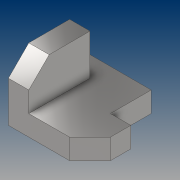
# Autodesk Inventor part: 10
Saved by Autodesk Inventor 2020.2 (Build 242310000, 310)
## iProperties
Created: 2020-09-17
Part Number: 10
Material: 鋼、碳鋼
Document SubType Name: Modeling
Designer: user
Density: 7.85 g/cm^3
Appearance: 半拋光
Mass: 149.15 g
Surface Area: 56.8284 cm^2
Volume: 19 cm^3
Author: user
Autodesk Inventor part; units mm, degrees
ref_plane "YZ Plane" through (0, 0, 0) normal (1, 0, 0) x (0, 1, 0)
ref_plane "XZ Plane" through (0, 0, 0) normal (0, 1, 0) x (-1, 0, 0)
ref_plane "XY Plane" through (0, 0, 0) normal (0, 0, 1) x (1, 0, 0)
sketch "草圖1" plane through (0, 0, 0) normal (0, 1, 0) x (-1, 0, 0)
  line L0 (0, 0) -> (-40, 0)
  line L1 (-40, 0) -> (-40, 40)
  line L2 (-40, 40) -> (0, 40)
  line L3 (0, 40) -> (0, 0)
  line L4 (-30, 0) -> (-30, 20)
  line L5 (-30, 20) -> (-40, 20)
  line L6 (-30, 40) -> (-40, 30)
  dimension "d0" = 40
  dimension "d1" = 40
  dimension "d2" = 10
  dimension "d3" = 20
  dimension "d4" = 10
  dimension "d5" = 10
  constraints: 14 end point, 3 point on line, 2 parallel, 2 perpendicular, 1 horizontal, 1 midpoint, 1 vertical
  measures "d0" distance of L0.start L0.end
  measures "d1" distance of L2.end L0.start
  measures "d2" distance between parallel lines of L1 L4
  measures "d3" distance of L4.start L4.end
  measures "d4" distance from line of L2 L6.end
  measures "d5" distance from line of L6.start L1
extrude "擠出1" add sketch "草圖1" along normal blind 10 contours L0 L4 L5 L1 L6 L2 L3
sketch "草圖2" plane through (0, 0, 0) normal (-1, 0, 0) x (0, 0, 1)
  line L0 (40, 10) -> (40, 0) projected
  line L1 (40, 0) -> (0, 0) projected
  line L2 (0, 0) -> (0, 10) projected
  line L3 (0, 10) -> (40, 10) projected
  line L4 (40, 10) -> (40, 20)
  line L5 (40, 20) -> (30, 30)
  line L6 (30, 30) -> (10, 30)
  line L7 (10, 30) -> (10, 10)
  line L8 (10, 10) -> (40, 10)
  dimension "d8" = 30
  dimension "d9" = 10
  dimension "d10" = 10
  dimension "d11" = 30
  constraints: 10 end point, 2 perpendicular, 1 collinear, 1 point on line, 1 vertical
  measures "d8" distance between parallel lines of L7 L4
  measures "d9" horizontal distance of L4.end L5.end
  measures "d10" horizontal distance of L4.end L5.end
  measures "d11" distance between parallel lines of L1 L6
extrude "擠出2" add sketch "草圖2" against normal blind 10 contours L3 L7 L6 L5 L4
equation "\"d10\" = d9"
